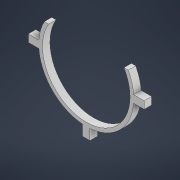
# Autodesk Inventor part: Clip_TestFitV1
Saved by Autodesk Inventor 2022 (Build 260153000, 153)
## iProperties
Created: 2023-05-05
Part Number: Clip_TestFitV1
Material: Generic
Document SubType Name: Modeling
Designer: User
Density: 1 g/cm^3
Appearance: Default
Author: User
Autodesk Inventor part; units mm, degrees
ref_plane "YZ Plane" through (0, 0, 0) normal (1, 0, 0) x (0, 1, 0)
ref_plane "XZ Plane" through (0, 0, 0) normal (0, 1, 0) x (-1, 0, 0)
ref_plane "XY Plane" through (0, 0, 0) normal (0, 0, 1) x (1, 0, 0)
sketch "Sketch1" plane through (0, 0, 0) normal (0, 0, 1) x (1, 0, 0)
  arc A0 (-25.4018, 15) -> (25.4018, 15) centre (0, 0) ccw
  line L0 (-28.2666, 15) -> (-25.4018, 15)
  line L1 (25.4018, 15) -> (28.2666, 15)
  line L2 (-39, 2.5) -> (-32, 2.5)
  line L3 (-32, -2.5) -> (-39, -2.5)
  line L4 (-39, -2.5) -> (-39, 2.5)
  line L5 (-32, 2.5) -> (-31.9022, 2.5)
  line L6 (-32, -2.5) -> (-31.9022, -2.5)
  line L7 (2.5, -32) -> (2.5, -39)
  line L8 (2.5, -39) -> (-2.5, -39)
  line L9 (-2.5, -39) -> (-2.5, -32)
  line L10 (-2.5, -32) -> (-2.5, -31.9022)
  line L11 (2.5, -32) -> (2.5, -31.9022)
  line L12 (32, 2.5) -> (39, 2.5)
  line L13 (39, 2.5) -> (39, -2.5)
  line L14 (39, -2.5) -> (32, -2.5)
  line L15 (32, 2.5) -> (31.9022, 2.5)
  line L16 (32, -2.5) -> (31.9022, -2.5)
  arc A1 (-28.2666, 15) -> (-31.9022, 2.5) centre (0, 0) ccw
  arc A2 (-31.9022, -2.5) -> (-2.5, -31.9022) centre (0, 0) ccw
  arc A3 (2.5, -31.9022) -> (31.9022, -2.5) centre (0, 0) ccw
  arc A4 (31.9022, 2.5) -> (28.2666, 15) centre (0, 0) ccw
  dimension "d18" = 59
  dimension "d41" = 7
  dimension "d42" = 5
  dimension "d43" = 5
  dimension "d44" = 7
  dimension "d45" = 7
  dimension "d46" = 5
  constraints: 34 end point, 10 point on circle, 7 horizontal, 5 centre point, 4 equal length, 2 vertical, 1 coincident, 1 perpendicular
  measures "d18" diameter of A0
  measures "d41" distance of L3.start L3.end
  measures "d42" distance of L2.end L3.start
  measures "d43" distance of L7.end L8.end
  measures "d44" distance of L7.start L7.end
  measures "d45" distance of L13.end L14.end
  measures "d46" distance of L12.end L13.end
extrude "Extrusion2" add sketch "Sketch1" along normal blind 5
body "Solid2"
